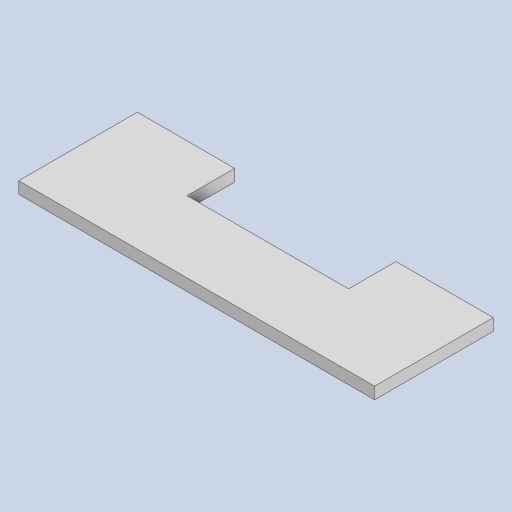
# Autodesk Inventor part: base
Saved by Autodesk Inventor 2023 (Build 270158000, 158)
## iProperties
Created: 2024-08-28
Part Number: base
Material: Generic
Document SubType Name: Modeling
Designer: kiyo
Density: 1 g/cm^3
Appearance: Default
Author: kiyo
Autodesk Inventor part; units mm, degrees
ref_plane "YZ Plane" through (0, 0, 0) normal (1, 0, 0) x (0, 1, 0)
ref_plane "XZ Plane" through (0, 0, 0) normal (0, 1, 0) x (-1, 0, 0)
ref_plane "XY Plane" through (0, 0, 0) normal (0, 0, 1) x (1, 0, 0)
sketch "スケッチ1" plane through (0, 0, 0) normal (0, 0, 1) x (1, 0, 0)
  line L0 (0, 0) -> (100, 0)
  line L1 (100, 0) -> (100, 300)
  line L2 (100, 300) -> (0, 300)
  line L3 (0, 300) -> (0, 0)
  line L4 (0, 218) -> (40, 218)
  line L5 (40, 218) -> (40, 82)
  line L6 (40, 82) -> (0, 82)
  line L7 (0, 82) -> (0, 218)
  point P0 (0, 150)
  point P1 (40, 150)
  point P2 (0, 82)
  dimension "d0" = 136
  dimension "d1" = 300
  dimension "d2" = 100
  dimension "d3" = 40
  dimension "d4" = 0
  constraints: 16 end point, 4 parallel, 2 horizontal, 2 midpoint, 2 perpendicular, 1 point on line
  measures "d0" distance of L4.end L5.end
  measures "d1" distance of L0.end L1.end
  measures "d2" distance of L0.start L0.end
  measures "d3" distance of L4.start L4.end
  measures "d4" vertical distance of point (0, 150) point (40, 150)
extrude "押し出し1" add sketch "スケッチ1" along normal blind 10 contours L3 L6 L5 L4 L2 L1 L0
